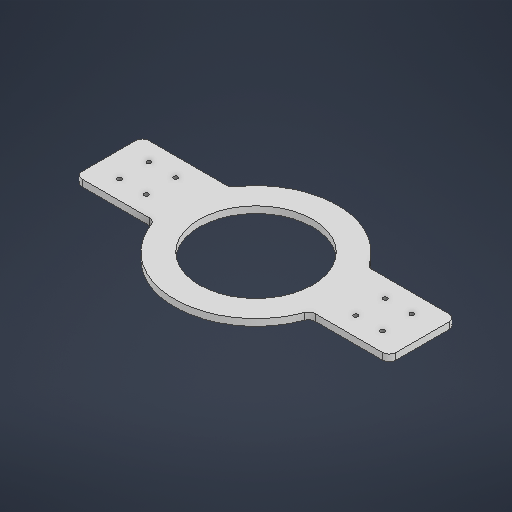
# Autodesk Inventor part: Head Thing (metal)
Saved by Autodesk Inventor 2025 (Build 290162000, 162)
## iProperties
Created: 2025-02-06
Part Number: Head Thing (metal)
Material: Generic
Document SubType Name: Modeling
Designer: mayhe
Density: 1 g/cm^3
Appearance: Default
Author: mayhe
Autodesk Inventor part; units mm, degrees
ref_plane "YZ Plane" through (0, 0, 0) normal (1, 0, 0) x (0, 1, 0)
ref_plane "XZ Plane" through (0, 0, 0) normal (0, 1, 0) x (-1, 0, 0)
ref_plane "XY Plane" through (0, 0, 0) normal (0, 0, 1) x (1, 0, 0)
sketch "Sketch1" plane through (0, 0, 0) normal (0, 1, 0) x (-1, 0, 0)
  circle A0 centre (0, 0) radius 42.5
  line L0 (-117.5, 17.713) -> (-117.5, -32.287)
  line L1 (117.5, -32.287) -> (117.5, 17.713)
  line L2 (-117.5, -32.287) -> (-51.7547, -32.287)
  line L3 (51.7547, -32.287) -> (117.5, -32.287)
  line L4 (117.5, 17.713) -> (58.3717, 17.713)
  line L5 (-58.3717, 17.713) -> (-117.5, 17.713)
  line L6 (117.5, 17.713) -> (63.9754, -2.1495) construction
  line L7 (-59.805, -14.1774) -> (-117.5, -32.287) construction
  line L8 (-117.5, 17.713) -> (-59.805, 12.2523) construction
  line L9 (63.9754, -28.5792) -> (117.5, -32.287) construction
  arc A1 (-51.7547, -32.287) -> (51.7547, -32.287) centre (0, 0) ccw
  arc A2 (58.3717, 17.713) -> (-58.3717, 17.713) centre (0, 0) ccw
  line L10 (0, 0) -> (0, -61)
  line L11 (0, 0) -> (0, 0)
  line L12 (0, 0) -> (0, -90.4875)
  dimension "d0" = 85
  dimension "d1" = 235
  dimension "d2" = 50
  dimension "d22" = 59.1283
  dimension "d23" = 59.1283
  dimension "d25" = 50
  dimension "d28" = 61
  dimension "d29" = 61
  constraints: 26 end point, 5 parallel, 5 point on circle, 3 centre point, 3 coincident, 3 horizontal, 2 perpendicular, 2 vertical, 1 point on line, 1 vertical alignment
  measures "d0" diameter of A0
  measures "d1" distance of L1.start L0.end
  measures "d2" distance of L0.end L0.start
  measures "d22" distance of L1.end L4.end
  measures "d23" distance of L5.start L0.start
  measures "d25" distance between parallel lines of L4 L3
  measures "d28" radius of A1
  measures "d29" radius of A2
extrude "Extrusion1" add sketch "Sketch1" along normal blind 5
sketch "Sketch2" plane through (0, 0, 0) normal (0, -1, 0) x (1, 0, 0)
  circle A0 centre (-98.5, -18.287) radius 2.5
  circle A1 centre (-98.5, 3.713) radius 2.5
  line L0 (-117.5, -32.287) -> (-117.5, 17.713) projected
  line L1 (-117.5, 17.713) -> (-58.3717, 17.713) projected
  line L2 (0, 0) -> (0, 61)
  arc A2 (58.3717, 17.713) -> (-58.3717, 17.713) centre (0, 0) ccw projected
  circle A3 centre (98.5, -18.287) radius 2.5
  circle A4 centre (98.5, 3.713) radius 2.5
  circle A5 centre (-78.5, -18.287) radius 2.5
  circle A6 centre (-78.5, 3.713) radius 2.5
  circle A7 centre (78.5, -18.287) radius 2.5
  circle A8 centre (78.5, 3.713) radius 2.5
  line L3 (-51.7547, -32.287) -> (-117.5, -32.287) projected
  dimension "d5" = 5
  dimension "d6" = 5
  dimension "d7" = 22
  dimension "d8" = 19
  dimension "d9" = 19
  dimension "d10" = 14
  dimension "d19" = 5
  dimension "d20" = 20
  dimension "d21" = 5
  dimension "d30" = 22
  dimension "d31" = 14
  dimension "d32" = 20
  constraints: 8 centre point, 5 symmetric about line, 2 end point, 1 point on circle, 1 vertical, 4 other
  measures "d5" diameter of A0
  measures "d6" diameter of A1
  measures "d7" distance of A0.centre A1.centre
  measures "d8" distance from line of L0 A0.centre
  measures "d9" distance from line of L0 A1.centre
  measures "d10" distance from line of L1 A1.centre
  measures "d19" diameter of A5
  measures "d20" distance of A5.centre A0.centre
  measures "d21" diameter of A6
  measures "d30" distance of A5.centre A6.centre
  measures "d31" distance from line of L3 A5.centre
  measures "d32" distance of A1.centre A6.centre
hole "Hole1" at (-98.5, 0, 3.713) at (-98.5, 0, -18.287) at (98.5, 0, 3.713) at (98.5, 0, -18.287) at (-78.5, 0, 3.713) at (-78.5, 0, -18.287) at (78.5, 0, -18.287) at (78.5, 0, 3.713) direction (0, 1, 0) diameter 3.242 depth 11.8 tip angle 118 thread size "M4x0.7" class "6H" standard "ANSI Metric M Profile"
fillet "Fillet1" radius 5 8 edges at (-51.7547, 2.5, -32.287) (-117.5, 2.5, -32.287) (-117.5, 2.5, 17.713) (51.7547, 2.5, -32.287) (117.5, 2.5, -32.287) (117.5, 2.5, 17.713) (58.3717, 2.5, 17.713) (-58.3717, 2.5, 17.713)
body "Solid1"
